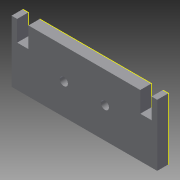
# Autodesk Inventor part: ex_holder_stopper
Saved by Autodesk Inventor 2014 SP1 (Build 180222100, 222)
## iProperties
Created: 2014-01-31
Part Number: ex_holder_stopper
Material: Wood (Birch)
Document SubType Name: Modeling
Designer: aoki
Density: 0.55 g/cm^3
Appearance: Birch - Natural Polished
Author: aoki
Autodesk Inventor part; units mm, degrees
ref_plane "YZ Plane" through (0, 0, 0) normal (1, 0, 0) x (0, 1, 0)
ref_plane "XZ Plane" through (0, 0, 0) normal (0, 1, 0) x (-1, 0, 0)
ref_plane "XY Plane" through (0, 0, 0) normal (0, 0, 1) x (1, 0, 0)
sketch "Sketch1" plane through (0, 0, 0) normal (0, 1, 0) x (-1, 0, 0)
  line L0 (35.5, -15) -> (-35.5, -15)
  line L1 (-35.5, -15) -> (-35.5, 15)
  line L2 (-35.5, 15) -> (35.5, 15)
  line L3 (35.5, 15) -> (35.5, -15)
  line L4 (35.5, -15) -> (-35.5, 15) construction
  line L5 (-35.5, -15) -> (35.5, 15) construction
  point P0 (0, 0)
  dimension "d0" = 71
  dimension "d5" = 30
  constraints: 12 end point, 2 midpoint, 2 parallel, 1 horizontal, 1 perpendicular
  measures "d0" distance of L1.end L2.end
  measures "d5" distance of L0.end L1.end
extrude "Extrusion1" add sketch "Sketch1" along normal blind 5.5
sketch "Sketch3" plane through (0, 5.5, 0) normal (0, 1, 0) x (1, 0, 0)
  line L0 (-35.5, -15) -> (35.5, -15) projected
  line L1 (0, 22.4425) -> (0, -29.6547) projected
  line L2 (-27.25, -15) -> (-32.75, -15)
  line L3 (-32.75, -15) -> (-32.75, -5)
  line L4 (-32.75, -5) -> (-27.25, -5)
  line L5 (-27.25, -5) -> (-27.25, -15)
  line L6 (-30, -0.7186) -> (-30, -17.2123)
  line L7 (27.25, -15) -> (32.75, -15)
  line L8 (32.75, -15) -> (32.75, -5)
  line L9 (32.75, -5) -> (27.25, -5)
  line L10 (27.25, -5) -> (27.25, -15)
  point P0 (0, 0)
  dimension "d6" = 5.5
  dimension "d7" = 10
  dimension "d8" = 30
  constraints: 18 end point, 4 symmetric about line, 3 parallel, 1 horizontal, 1 perpendicular, 1 point on line, 1 other
  measures "d6" distance of L3.end L4.end
  measures "d7" distance of L2.end L3.end
  measures "d8" distance between parallel lines of L1 L6
extrude "Extrusion2" cut sketch "Sketch3" against normal through all
sketch "Sketch4" plane through (0, 5.5, 0) normal (0, 1, 0) x (1, 0, 0)
  line L0 (-27.25, -5) -> (-27.25, -15) projected
  line L1 (-27.25, -15) -> (27.25, -15) projected
  line L2 (27.25, -15) -> (27.25, -5) projected
  line L3 (27.25, -5) -> (32.75, -5) projected
  line L4 (32.75, -5) -> (32.75, -15) projected
  line L5 (32.75, -15) -> (35.5, -15) projected
  line L6 (35.5, -15) -> (35.5, 15) projected
  line L7 (35.5, 15) -> (-35.5, 15) projected
  line L8 (-35.5, 15) -> (-35.5, -15) projected
  line L9 (-35.5, -15) -> (-32.75, -15) projected
  line L10 (-32.75, -15) -> (-32.75, -5) projected
  line L11 (-32.75, -5) -> (-27.25, -5) projected
  point P0 (0, 0)
sketch "Sketch5" plane through (0, 0, 0) normal (0, -1, 0) x (1, 0, 0)
  line L0 (-49.7, 0) -> (49.7, 0) projected
  line L1 (0, -21) -> (0, 21) projected
  circle A0 centre (-10, 0) radius 2
  circle A1 centre (10, 0) radius 2
  point P0 (0, 0)
  dimension "d11" = 4
  dimension "d12" = 20
  constraints: 2 centre point, 1 point on line, 1 symmetric about line, 1 other
  measures "d11" diameter of A0
  measures "d12" distance of A1.centre A0.centre
extrude "Extrusion3" cut sketch "Sketch5" against normal through all
equation "\"d1\" = Wt"
equation "\"d6\" = Wt"
equation "\"Wt\" = 5.5"
body "Solid1"
